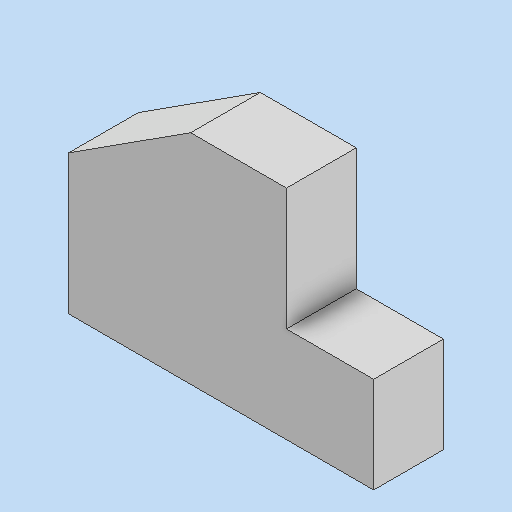
# Autodesk Inventor part: Peça2
Saved by Autodesk Inventor 2025.3 (Build 293356000, 356)
## iProperties
Created: 2025-10-09
Part Number: Peça2
Material: Genérico
Document SubType Name: Modeling
Designer: gabriel.bispo
Density: 1 g/cm^3
Appearance: Padrão
Author: gabriel.bispo
Autodesk Inventor part; units mm, degrees
ref_plane "YZ Plane" through (0, 0, 0) normal (1, 0, 0) x (0, 1, 0)
ref_plane "XZ Plane" through (0, 0, 0) normal (0, 1, 0) x (-1, 0, 0)
ref_plane "XY Plane" through (0, 0, 0) normal (0, 0, 1) x (1, 0, 0)
sketch "Esboço1" plane through (0, 0, 0) normal (0, 0, 1) x (1, 0, 0)
  line L0 (0, 0) -> (35, 0)
  line L1 (35, 0) -> (35, 11)
  line L2 (35, 11) -> (25, 11)
  line L3 (25, 11) -> (25, 25)
  line L4 (25, 25) -> (14, 25)
  line L5 (14, 25) -> (0, 16)
  line L6 (0, 16) -> (0, 0)
  dimension "d0" = 35
  dimension "d1" = 11
  dimension "d2" = 14
  dimension "d3" = 10
  dimension "d4" = 9
  dimension "d5" = 11
  constraints: 14 end point, 4 perpendicular, 1 horizontal, 1 parallel
  measures "d0" distance of L0.start L0.end
  measures "d1" distance of L0.end L1.end
  measures "d2" distance between parallel lines of L2 L4
  measures "d3" distance between parallel lines of L1 L3
  measures "d4" vertical distance of L4.end L5.end
  measures "d5" distance of L3.end L4.end
extrude "Extrusão1" add sketch "Esboço1" along normal blind 8
